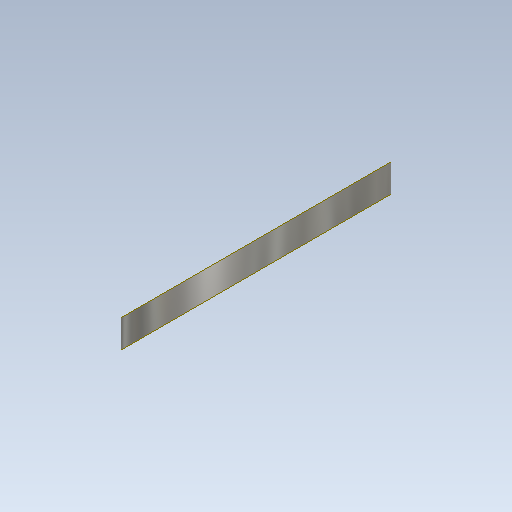
# Autodesk Inventor part: Część1
Saved by Autodesk Inventor 2020 (Build 240168000, 168)
## iProperties
Created: 2019-05-27
Part Number: Część1
Material: Srebrny
Document SubType Name: Modeling
Designer: barto
Density: 10.49 g/cm^3
Appearance: Srebrny
Author: barto
Autodesk Inventor part; units mm, degrees
ref_plane "YZ Plane" through (0, 0, 0) normal (1, 0, 0) x (0, 1, 0)
ref_plane "XZ Plane" through (0, 0, 0) normal (0, 1, 0) x (-1, 0, 0)
sketch "Szkic1" plane through (0, 0, 0) normal (0, 1, 0) x (-1, 0, 0)
  circle A0 centre (0, 0) radius 17
  dimension "d0" = 34
  constraints: 1 centre point, 1 coincident
  measures "d0" diameter of A0
extrude "Wyciągnięcie proste1" add sketch "Szkic1" along normal blind 39
ref_plane "Płaszczyzna konstrukcyjna1" through (0, 0, 26) normal (0, 0, 1) x (1, 0, 0)
sketch "Szkic3" plane through (0, 0, 26) normal (0, 0, 1) x (1, 0, 0)
  line L0 (17, 39) -> (-17, 39) projected
  line L1 (-17, 39) -> (17, 39)
  line L2 (17, 39) -> (-18.3291, 3.6709)
  line L3 (-18.3291, 3.6709) -> (-17, 39)
  line L4 (-17, 0) -> (17, 0) projected
  line L5 (17, 0) -> (-17, 0)
  line L6 (-17, 0) -> (20.0902, 37.0902)
  line L7 (20.0902, 37.0902) -> (17, 0)
  point P0 (0, 0)
  dimension "d4" = 45
  dimension "d5" = 45
  constraints: 12 end point, 1 collinear, 1 horizontal
  measures "d4" angle of L1 L2
  measures "d5" angle of L5 L6
extrude "Wyciągnięcie proste2" cut sketch "Szkic3" against normal blind 53.75
